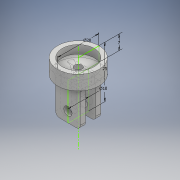
# Autodesk Inventor part: piston
Saved by Autodesk Inventor 2018 (Build 220112000, 112)
## iProperties
Created: 2025-02-23
Part Number: piston
Material: Generic
Document SubType Name: Modeling
Designer: neo
Density: 1 g/cm^3
Appearance: Default
Author: neo
Autodesk Inventor part; units mm, degrees
ref_plane "YZ Plane" through (0, 0, 0) normal (1, 0, 0) x (0, 1, 0)
ref_plane "XZ Plane" through (0, 0, 0) normal (0, 1, 0) x (-1, 0, 0)
ref_plane "XY Plane" through (0, 0, 0) normal (0, 0, 1) x (1, 0, 0)
sketch "Sketch1" plane through (0, 0, 0) normal (1, 0, 0) x (0, 1, 0)
  line L0 (0, 21.5591) -> (0, -21.8295)
  line L1 (10, 16.8036) -> (0, 16.8036)
  line L2 (0, 16.8036) -> (0, 9.8036)
  line L3 (0, 9.8036) -> (10, 9.8036)
  line L4 (10, 9.8036) -> (10, 16.8036)
  line L5 (5, 9.8036) -> (0, 9.8036)
  line L6 (0, 9.8036) -> (0, -8.1964)
  line L7 (0, -8.1964) -> (5, -8.1964)
  line L8 (5, -8.1964) -> (5, 9.8036)
  line L9 (-5, 9.8036) -> (0, 9.8036)
  line L10 (0, -8.1964) -> (-5, -8.1964)
  line L11 (-5, -8.1964) -> (-5, 9.8036)
  point P0 (0, 0)
  dimension "d0" = 20
  dimension "d1" = 7
  dimension "d5" = 10
  dimension "d7" = 25
  constraints: 24 end point, 4 parallel, 2 horizontal, 2 perpendicular, 2 point on line, 2 symmetric about line, 1 midpoint, 1 vertical
  measures "d0" diameter of L4 L0
  measures "d1" distance of L3.end L1.start
  measures "d5" diameter of L8 L0
  measures "d7" distance between parallel lines of L1 L7
revolve "Revolution1" add sketch "Sketch1" angle 360 about axis through (0, 0, 21.5591) along (0, 0, -1) contours L1 L4 L3 L0
extrude "Extrusion1" add sketch "Sketch1" along normal mid plane 12 contours L3 L8 L7 L0 | L0 L10 L11 L9
hole "Hole1" at (0, 0, 16.8036) direction (0, 0, -1) diameter 3.5 end through all counterbore diameter 15.5 counterbore depth 4
ref_plane "Work Plane1" through (0, 0, 9.8036) normal (0, 0, 1) x (1, 0, 0)
sketch "Sketch2" plane through (6, 5, -8.1964) normal (0, 0, -1) x (-1, 0, 0)
  circle A0 centre (6, -5) radius 1.75 projected
  line L0 (6, -5) -> (18.5307, -5)
  line L1 (15.8465, -2.5) -> (-5.7871, -2.5)
  line L2 (-5.7871, -2.5) -> (-5.7871, -7.5)
  line L3 (-5.7871, -7.5) -> (15.8465, -7.5)
  line L4 (15.8465, -7.5) -> (15.8465, -2.5)
  dimension "d20" = 5
  constraints: 10 end point, 2 horizontal, 2 parallel, 1 perpendicular, 1 other
  measures "d20" distance between parallel lines of L1 L3
extrude "Extrusion2" cut sketch "Sketch2" against normal up to surface (18 mm away)
sketch "Sketch3" plane through (0, 0, 9.8036) normal (0, 0, -1) x (-1, 0, 0)
  line L0 (-4, 4) -> (4, 4)
  line L1 (4, 4) -> (4, -4)
  line L2 (4, -4) -> (-4, -4)
  line L3 (-4, -4) -> (-4, 4)
  line L4 (0, 0) -> (0, 10) projected
  circle A0 centre (0, 0) radius 1.75 projected
  line L5 (0, 0) -> (-11.0224, 0)
  dimension "d23" = 8
  constraints: 10 end point, 2 horizontal, 2 parallel, 2 perpendicular, 2 other
  measures "d23" distance of L0.end L1.end
extrude "Extrusion3" cut sketch "Sketch3" along normal blind 4 contours L0 L4 A0 L5 L3 | L0 L1 L2 L3 L5 A0 L4
sketch "Sketch4" plane through (-6, -5, -8.1964) normal (0, -1, 0) x (1, 0, 0)
  line L0 (0, 18) -> (12, 18) projected
  line L1 (0, 0) -> (0, 18) projected
  line L2 (0, 0) -> (12, 0) projected
  line L3 (12, 18) -> (12, 0) projected
  circle A0 centre (6, 5) radius 2
  point P0 (6, 8.1964)
  dimension "d26" = 5
  dimension "d27" = 4
  constraints: 1 centre point
  measures "d26" distance from line of L2 A0.centre
  measures "d27" diameter of A0
extrude "Extrusion4" cut sketch "Sketch4" against normal through all contours A0
fillet "Fillet1" radius 2 2 edges at (6, -3.75, 9.8036) (6, 3.75, 9.8036)
fillet "Fillet1" radius 2 2 edges at (-6, -3.75, 9.8036) (-6, 3.75, 9.8036)
fillet "Fillet2" radius 2 4 edges at (6, -3.75, -8.1964) (-6, -3.75, -8.1964) (-6, 3.75, -8.1964) (6, 3.75, -8.1964)
body "Solid1"
